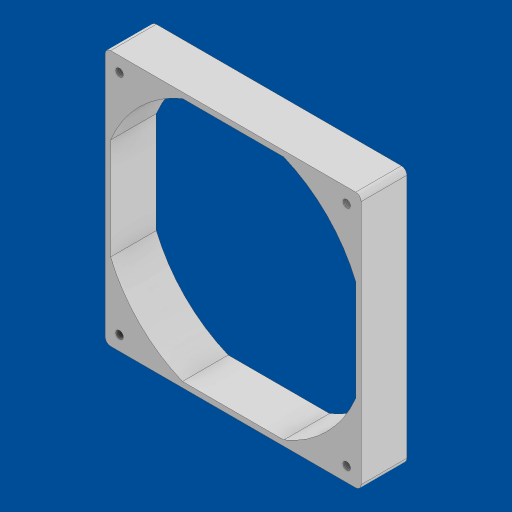
# Autodesk Inventor part: nf-a14
Saved by Autodesk Inventor 2023.2 (Build 272271000, 271)
## iProperties
Created: 2023-09-04
Part Number: nf-a14
Material: Generic
Document SubType Name: Modeling
Designer: agmlego
Mass: 96.7829 g
Surface Area: 335.607 cm^2
Volume: 96.7829 cm^3
Density: 1 g/cm^3
Appearance: Default
Author: agmlego
Autodesk Inventor part; units mm, degrees
ref_plane "YZ Plane" through (0, 0, 0) normal (1, 0, 0) x (0, 1, 0)
ref_plane "XZ Plane" through (0, 0, 0) normal (0, 1, 0) x (-1, 0, 0)
ref_plane "XY Plane" through (0, 0, 0) normal (0, 0, 1) x (1, 0, 0)
sketch "Sketch1" plane through (0, 0, 0) normal (0, 0, 1) x (1, 0, 0)
  line L0 (-67, -70) -> (67, -70)
  line L1 (70, -67) -> (70, 67)
  line L2 (67, 70) -> (-67, 70)
  line L3 (-70, 67) -> (-70, -67)
  line L4 (-70, -70) -> (70, 70) construction
  line L5 (70, -70) -> (-70, 70) construction
  arc A0 (-67, 70) -> (-70, 67) centre (-67, 67) ccw
  arc A1 (-70, -67) -> (-67, -70) centre (-67, -67) ccw
  arc A2 (67, -70) -> (70, -67) centre (67, -67) ccw
  arc A3 (70, 67) -> (67, 70) centre (67, 67) ccw
  line L6 (-62.1, -62.1) -> (62.1, -62.1) construction
  line L7 (62.1, -62.1) -> (62.1, 62.1) construction
  line L8 (62.1, 62.1) -> (-62.1, 62.1) construction
  line L9 (-62.1, 62.1) -> (-62.1, -62.1) construction
  line L10 (-62.1, -62.1) -> (62.1, 62.1) construction
  line L11 (62.1, -62.1) -> (-62.1, 62.1) construction
  line L12 (-27.6993, 67) -> (27.6993, 67)
  line L13 (67, 27.6993) -> (67, -27.6993)
  line L14 (27.6993, -67) -> (-27.6993, -67)
  line L15 (-67, -27.6993) -> (-67, 27.6993)
  arc A4 (67, 27.6993) -> (27.6993, 67) centre (0, 0) ccw
  arc A5 (27.6993, -67) -> (67, -27.6993) centre (0, 0) ccw
  arc A6 (-27.6993, 67) -> (-67, 27.6993) centre (0, 0) ccw
  arc A7 (-67, -27.6993) -> (-27.6993, -67) centre (0, 0) ccw
  point P0 (0, 0)
  point P1 (51.2652, -51.2652)
  point P2 (-51.2652, 51.2652)
  dimension "d0" = 140
  dimension "d1" = 140
  dimension "d2" = 3
  dimension "d3" = 124.2
  dimension "d4" = 124.2
  dimension "d6" = 145
  dimension "d7" = 134
  constraints: 32 end point, 18 point on circle, 8 centre point, 8 point on line, 8 tangent, 6 equal radius, 5 coincident, 5 perpendicular, 4 midpoint, 4 parallel, 3 equal length, 3 horizontal
  measures "d0" distance of L5.end L4.end
  measures "d1" distance of L4.end L5.start
  measures "d2" radius of A0
  measures "d3" distance of L8.end L7.end
  measures "d4" distance of L7.end L6.end
  measures "d6" distance of point (51.265, -51.265) point (-51.265, 51.265)
  measures "d7" distance between parallel lines of L14 L12
extrude "Extrusion1" add sketch "Sketch1" along normal mid plane 25
hole "Hole1" at (-62.1, 62.1, 0) at (62.1, 62.1, 0) at (62.1, -62.1, 0) at (-62.1, -62.1, 0) direction (0, 0, 1) diameter 4.134 end through all thread size "M5x0.8" class "6H" standard "ANSI Metric M Profile"
body "Solid1"
